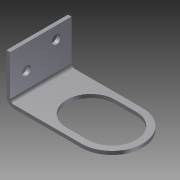
# Autodesk Inventor part: 13536
Saved by Autodesk Inventor 2014 (Build 180170000, 170)
## iProperties
Category: Pneumatics
Company: Autodesk, Inc.
Shininess: 64.0
Length Units: 11269
Angle Units: 11279
Time Units: 11290
Mass Units: 11283
Length Display Precision: 3
Angle Display Precision: 2
Compacted: True
Part Number: 13536
Document SubType Name: Sheet Metal
Created: 2011-11-10
Manufacturer: Standard
Standards Organization: Custom
Density: 1 g/cm^3
Project: FIRST
Description: Bracket for Secondary Regulator
Vendor: Monnier
Sheet Metal Rule: Default
Catalog Web Link: http://www.monnier.com/M98-Access.pdf
Material: Generic
Appearance: Default
Density: 0.0
Volumn: 0.0
Area: 0.0
PropertySet Name: Model Information
Control State: 0
Master: False
Checked Out: False
Title: Bracket - Secondary Regulator
Author: Autodesk, Inc.
Autodesk Inventor part; units mm, degrees
ref_plane "YZ Plane" through (0, 0, 0) normal (1, 0, 0) x (0, 1, 0)
ref_plane "XZ Plane" through (0, 0, 0) normal (0, 1, 0) x (-1, 0, 0)
ref_plane "XY Plane" through (0, 0, 0) normal (0, 0, 1) x (1, 0, 0)
sketch "Sketch1" plane through (0, 0, 0) normal (0, 0, 1) x (1, 0, 0)
  line L0 (-44, 19) -> (0, 19)
  line L1 (0, -19) -> (-44, -19)
  line L2 (-44, -19) -> (-44, 19)
  arc A0 (0, -19) -> (0, 19) centre (0, 0) ccw
  arc A1 (0, -15) -> (0, 15) centre (0, 0) ccw
  arc A2 (-13, 15) -> (-13, -15) centre (-13, 0) ccw
  line L3 (0, 15) -> (-13, 15)
  line L4 (0, -15) -> (-13, -15)
  dimension "d0" = 38
  dimension "d1" = 63
  dimension "d2" = 4
  dimension "d3" = 43
  measures "d0" distance between parallel lines of L1 L0
  measures "d2" distance between parallel lines of L0 L3
extrude "Plate1" add sketch "Sketch1" along normal blind 2.2
sketch "Sketch2" plane through (-44, -19, 2.2) normal (1, 0, 0) x (0, 1, 0)
  line L0 (0, 0) -> (38, 0)
  line L1 (38, 0) -> (38, 27)
  line L2 (38, 27) -> (0, 27)
  line L3 (0, 27) -> (0, 0)
  constraints: 6 end point, 1 horizontal, 1 perpendicular, 1 vertical
sheet face with bend "Flange1" sketch "Sketch2" thickness 2.2 toward (-1, 0, 0) bend radius 2.2 relief tear relief width 2.2 relief depth 1.1
bend "Bend1"
sketch "Sketch3" plane through (-46.2, -19, 29.2) normal (-1, 0, 0) x (0, 0, 1)
  line L0 (-24.8, 38) -> (-24.8, 0) projected
  line L1 (0, 0) -> (-24.8, 0) projected
  line L2 (0, 38) -> (0, 0) projected
  line L3 (-24.8, 38) -> (0, 38) projected
  circle A0 centre (-7.5, 28.5) radius 2.75
  circle A1 centre (-15, 10) radius 2.75
  dimension "d12" = 5.5
  dimension "d13" = 9.5
  dimension "d14" = 7.5
  dimension "d15" = 10
  dimension "d16" = 15
  constraints: 2 centre point, 1 equal radius
  measures "d12" diameter of A0
  measures "d13" distance from line of L3 A0.centre
  measures "d14" distance from line of L2 A0.centre
  measures "d15" distance from line of L1 A1.centre
  measures "d16" distance from line of L2 A1.centre
extrude "Cut1" cut sketch "Sketch3" against normal blind 2.2 contours A0 | A1
equation "\"d17\" = Thickness"
equation "\"d5\" = BendReliefWidth"
equation "\"d7\" = MinimumRemnant"
equation "\"d11\" = BendRadius"
equation "\"d6\" = BendReliefDepth"
equation "\"d8\" = BendRadius"
equation "\"BendRadius\" = Thickness"
equation "\"BendReliefWidth\" = Thickness"
equation "\"BendReliefDepth\" = 0.5 * Thickness"
equation "\"CornerReliefSize\" = 4 * Thickness"
equation "\"MinimumRemnant\" = 2 * Thickness"
equation "\"TransitionRadius\" = BendRadius"
equation "\"d4\" = BendRadius"
equation "\"JacobiRadiusSize\" = Thickness"
equation "\"GapSize\" = Thickness"
equation "\"Thickness\" = 2.2"
body "Solid1"
